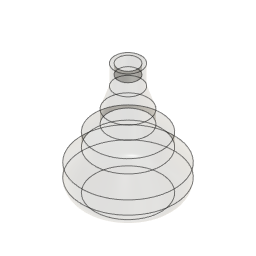
Qatest-MillTurn New Features (Autodesk Fusion 360 design; units mm, degrees)
Autodesk Fusion 360 part; units mm, degrees
sketch "Sketch1" plane through (0, 0, 0) normal (0, 1, 0) x (1, 0, 0)
  line L0 (70, -20) -> (70, -40)
  line L1 (70, -40) -> (50, -60)
  line L2 (50, -60) -> (50, -80)
  line L3 (50, -80) -> (30, -90)
  line L4 (30, -90) -> (30, -110)
  line L5 (30, -110) -> (20, -140)
  line L6 (20, -140) -> (20, -170)
  line L7 (20, -170) -> (0, -170)
  line L8 (0, -170) -> (0, 0)
  line L9 (0, 0) -> (50, 0)
  arc A0 (70, -20) -> (50, 0) centre (50, -20) ccw
  dimension "d3" = 20
  constraint vertical L0
  constraint parallel L0 L2
  constraint parallel L2 L4
  constraint parallel L4 L6
  constraint perpendicular L6 L7
  constraint coincident L8.end L9.start
  constraint perpendicular L7 L8
  constraint perpendicular L8 L9
  constraint tangent L9 A0
  constraint tangent L0 A0
  measures "d3" radius of A0
revolve "Revolve1" add sketch "Sketch1" angle 360 about axis through (0, 0, 170) along (0, 0, -1)
sketch "Sketch2" plane through (0, 0, 170) normal (0, 0, 1) x (-1, 0, 0)
  circle A0 centre (0, 0) radius 20
  circle A1 centre (0, 0) radius 15
  dimension "d4" = 30
  constraint concentric A0 A1
  measures "d4" diameter of A1
extrude "Extrude1" cut sketch "Sketch2" against normal blind 15 contours A1
